Autodesk Inventor part; units mm, degrees
(part 2 of 2)
sketch "Sketch3" plane through (0.0295, 41.5, 0) normal (0, 1, 0) x (1, 0, 0)
  line L0 (1770.5478, -680) -> (1790.5478, -680)
  line L1 (1790.5478, -640) -> (1770.5478, -640)
  line L2 (1790.5478, -620) -> (1790.5478, -640)
  line L3 (1770.5478, -640) -> (1770.5478, -620)
  line L4 (1770.5478, -620) -> (1790.5478, -620)
  line L5 (1790.5478, -680) -> (1790.5478, -700)
  line L6 (1770.5478, -700) -> (1770.5478, -680)
  line L7 (1790.5478, -700) -> (1770.5478, -700)
  line L8 (1770.5478, -740) -> (1790.5478, -740)
  line L9 (1790.5478, -740) -> (1790.5478, -760)
  line L10 (1790.5478, -760) -> (1770.5478, -760)
  line L11 (1770.5478, -760) -> (1770.5478, -740)
  line L12 (1790.5478, -580) -> (1770.5478, -580)
  line L13 (1770.5478, -580) -> (1770.5478, -560)
  line L14 (1770.5478, -560) -> (1790.5478, -560)
  line L15 (1790.5478, -340) -> (1770.5478, -340)
  line L16 (1790.5478, -320) -> (1790.5478, -340)
  line L17 (1770.5478, -340) -> (1770.5478, -320)
  line L18 (1770.5478, -320) -> (1790.5478, -320)
  line L19 (1790.5478, -280) -> (1770.5478, -280)
  line L20 (1770.5478, -280) -> (1770.5478, -260)
  line L21 (1770.5478, -260) -> (1790.5478, -260)
  line L22 (1790.5478, -260) -> (1790.5478, -280)
  line L23 (1790.5478, -560) -> (1790.5478, -580)
  line L24 (1770.5478, -520) -> (1770.5478, -500)
  line L25 (1770.5478, -500) -> (1790.5478, -500)
  line L26 (1790.5478, -500) -> (1790.5478, -520)
  line L27 (1790.5478, -520) -> (1770.5478, -520)
  line L28 (1770.5478, -460) -> (1770.5478, -440)
  line L29 (1790.5478, -460) -> (1770.5478, -460)
  line L30 (1770.5478, -440) -> (1790.5478, -440)
  line L31 (1790.5478, -400) -> (1770.5478, -400)
  line L32 (1770.5478, -400) -> (1770.5478, -380)
  line L33 (1790.5478, -380) -> (1790.5478, -400)
  line L34 (1790.5478, -440) -> (1790.5478, -460)
  line L35 (1790.5478, -220) -> (1770.5478, -220)
  line L36 (1770.5478, -220) -> (1770.5478, -200)
  line L37 (1770.5478, -200) -> (1790.5478, -200)
  line L38 (1790.5478, -200) -> (1790.5478, -220)
  line L39 (1770.5478, -380) -> (1790.5478, -380)
  line L40 (1790.5478, -100) -> (1770.5478, -100)
  line L41 (1790.5478, -80) -> (1790.5478, -100)
  line L42 (1770.5478, -100) -> (1770.5478, -80)
  line L43 (1770.5478, -80) -> (1790.5478, -80)
  line L44 (1790.5478, -40) -> (1770.5478, -40)
  line L45 (1770.5478, -20) -> (1790.5478, -20)
  line L46 (1790.5478, -20) -> (1790.5478, -40)
  line L47 (1770.5478, -40) -> (1770.5478, -20)
  line L48 (1790.5478, -160) -> (1770.5478, -160)
  line L49 (1790.5478, -140) -> (1790.5478, -160)
  line L50 (1770.5478, -160) -> (1770.5478, -140)
  line L51 (1770.5478, -140) -> (1790.5478, -140)
  line L52 (1938.8211, -400) -> (1938.8211, -380)
  line L53 (1958.8211, -400) -> (1938.8211, -400)
  line L54 (1958.8211, -380) -> (1958.8211, -400)
  line L55 (1938.8211, -380) -> (1958.8211, -380)
  line L56 (1938.8211, -340) -> (1938.8211, -320)
  line L57 (1958.8211, -340) -> (1938.8211, -340)
  line L58 (1958.8211, -320) -> (1958.8211, -340)
  line L59 (1938.8211, -320) -> (1958.8211, -320)
  line L60 (1958.8211, -280) -> (1938.8211, -280)
  line L61 (1958.8211, -260) -> (1958.8211, -280)
  line L62 (1938.8211, -280) -> (1938.8211, -260)
  line L63 (1938.8211, -260) -> (1958.8211, -260)
  line L64 (1958.8211, -220) -> (1938.8211, -220)
  line L65 (1958.8211, -200) -> (1958.8211, -220)
  line L66 (1938.8211, -200) -> (1958.8211, -200)
  line L67 (1938.8211, -220) -> (1938.8211, -200)
  line L68 (1938.8211, -100) -> (1938.8211, -80)
  line L69 (1958.8211, -80) -> (1958.8211, -100)
  line L70 (1958.8211, -100) -> (1938.8211, -100)
  line L71 (1938.8211, -160) -> (1938.8211, -140)
  line L72 (1938.8211, -140) -> (1958.8211, -140)
  line L73 (1958.8211, -160) -> (1938.8211, -160)
  line L74 (1958.8211, -140) -> (1958.8211, -160)
  line L75 (1938.8211, -80) -> (1958.8211, -80)
  line L76 (1958.8211, -40) -> (1938.8211, -40)
  line L77 (1958.8211, -20) -> (1958.8211, -40)
  line L78 (1938.8211, -20) -> (1958.8211, -20)
  line L79 (1938.8211, -40) -> (1938.8211, -20)
  line L80 (1958.8211, -520) -> (1938.8211, -520)
  line L81 (1938.8211, -520) -> (1938.8211, -500)
  line L82 (1958.8211, -500) -> (1958.8211, -520)
  line L83 (1938.8211, -500) -> (1958.8211, -500)
  line L84 (1958.8211, -460) -> (1938.8211, -460)
  line L85 (1958.8211, -440) -> (1958.8211, -460)
  line L86 (1938.8211, -440) -> (1958.8211, -440)
  line L87 (1938.8211, -460) -> (1938.8211, -440)
  line L88 (1958.8211, -640) -> (1938.8211, -640)
  line L89 (1938.8211, -560) -> (1958.8211, -560)
  line L90 (1938.8211, -580) -> (1938.8211, -560)
  line L91 (1958.8211, -560) -> (1958.8211, -580)
  line L92 (1958.8211, -580) -> (1938.8211, -580)
  line L93 (1938.8211, -620) -> (1958.8211, -620)
  line L94 (1938.8211, -640) -> (1938.8211, -620)
  line L95 (1958.8211, -620) -> (1958.8211, -640)
  line L96 (1938.8211, -760) -> (1938.8211, -740)
  line L97 (1938.8211, -700) -> (1938.8211, -680)
  line L98 (1938.8211, -680) -> (1958.8211, -680)
  line L99 (1958.8211, -680) -> (1958.8211, -700)
  line L100 (1958.8211, -700) -> (1938.8211, -700)
  line L101 (1938.8211, -740) -> (1958.8211, -740)
  line L102 (1958.8211, -740) -> (1958.8211, -760)
  line L103 (1958.8211, -760) -> (1938.8211, -760)
  point P0 (-0.0295, 0)
  point P1 (1780.5478, -640)
  point P2 (1780.5478, -700)
  point P3 (1780.5478, -760)
  point P4 (1780.5478, -740)
  point P5 (1780.5478, -580)
  point P6 (1780.5478, -340)
  point P7 (1780.5478, -280)
  point P8 (1780.5478, -520)
  point P9 (1780.5478, -500)
  point P10 (1780.5478, -460)
  point P11 (1780.5478, -400)
  point P12 (1780.5478, -220)
  point P13 (1780.5478, -40)
  point P14 (1780.5478, -160)
  point P15 (1780.5478, -100)
  point P16 (1948.8211, -400)
  point P17 (1948.8211, -340)
  point P18 (1948.8211, -280)
  point P19 (1948.8211, -220)
  point P20 (1948.8211, -100)
  point P21 (1948.8211, -160)
  point P22 (1948.8211, -40)
  point P23 (1948.8211, -520)
  point P24 (1948.8211, -500)
  point P25 (1948.8211, -460)
  point P26 (1948.8211, -640)
  point P27 (1948.8211, -580)
  point P28 (1948.8211, -700)
  point P29 (1948.8211, -760)
  point P30 (1948.8211, -740)
  dimension "d459" = 20
  dimension "d460" = 20
  dimension "d461" = 20
  dimension "d462" = 20
  dimension "d463" = 20
  dimension "d464" = 20
  dimension "d465" = 20
  dimension "d466" = 20
  dimension "d467" = 20
  dimension "d468" = 20
  dimension "d469" = 20
  dimension "d470" = 20
  dimension "d471" = 20
  dimension "d472" = 20
  dimension "d473" = 20
  dimension "d474" = 20
  dimension "d475" = 20
  dimension "d476" = 20
  dimension "d477" = 20
  dimension "d478" = 20
  dimension "d479" = 20
  dimension "d480" = 20
  dimension "d481" = 40
  dimension "d482" = 40
  dimension "d483" = 40
  dimension "d484" = 40
  dimension "d485" = 40
  dimension "d486" = 40
  dimension "d487" = 40
  dimension "d488" = 40
  dimension "d489" = 40
  dimension "d490" = 20
  dimension "d491" = 20
  dimension "d492" = 40
  dimension "d493" = 20
  dimension "d494" = 20
  dimension "d495" = 40
  dimension "d496" = 20
  dimension "d497" = 20
  dimension "d498" = 20
  dimension "d499" = 20
  dimension "d500" = 20
  dimension "d501" = 20
  dimension "d502" = 20
  dimension "d503" = 20
  dimension "d504" = 20
  dimension "d505" = 20
  dimension "d506" = 20
  dimension "d507" = 20
  dimension "d508" = 20
  dimension "d509" = 20
  dimension "d510" = 20
  dimension "d511" = 20
  dimension "d512" = 20
  dimension "d513" = 20
  dimension "d514" = 20
  dimension "d515" = 20
  dimension "d516" = 20
  dimension "d517" = 20
  dimension "d518" = 40
  dimension "d519" = 40
  dimension "d520" = 40
  dimension "d521" = 40
  dimension "d522" = 40
  constraints: 208 end point, 52 parallel, 30 midpoint, 26 horizontal, 26 perpendicular
  measures "d459" distance from line of point (1780.548, -40) L45
  measures "d460" distance between parallel lines of L46 L47
  measures "d461" distance from line of point (1780.548, -100) L43
  measures "d462" distance between parallel lines of L41 L42
  measures "d463" distance from line of point (1780.548, -160) L51
  measures "d464" distance between parallel lines of L49 L50
  measures "d465" distance from line of point (1780.548, -220) L37
  measures "d466" distance between parallel lines of L38 L36
  measures "d467" distance from line of point (1780.548, -400) L39
  measures "d468" distance between parallel lines of L33 L32
  measures "d469" distance from line of point (1780.548, -460) L30
  measures "d470" distance between parallel lines of L34 L28
  measures "d471" distance from line of point (1780.548, -520) L25
  measures "d472" distance between parallel lines of L26 L24
  measures "d473" distance from line of point (1780.548, -580) L14
  measures "d474" distance between parallel lines of L23 L13
  measures "d475" distance from line of point (1780.548, -640) L4
  measures "d476" distance between parallel lines of L2 L3
  measures "d477" distance from line of point (1780.548, -700) L0
  measures "d478" distance between parallel lines of L5 L6
  measures "d479" distance from line of point (1780.548, -760) L8
  measures "d480" distance between parallel lines of L9 L11
  measures "d481" distance between parallel lines of L43 L44
  measures "d482" distance between parallel lines of L51 L40
  measures "d483" distance between parallel lines of L37 L48
  measures "d484" distance from line of point (1780.548, -740) L7
  measures "d485" distance between parallel lines of L0 L1
  measures "d486" distance between parallel lines of L4 L12
  measures "d487" distance between parallel lines of L14 L27
  measures "d488" distance from line of point (1780.548, -500) L29
  measures "d489" distance between parallel lines of L31 L30
  measures "d490" distance from line of point (1780.548, -280) L21
  measures "d491" distance between parallel lines of L22 L20
  measures "d492" distance between parallel lines of L21 L35
  measures "d493" distance from line of point (1780.548, -340) L18
  measures "d494" distance between parallel lines of L16 L17
  measures "d495" distance between parallel lines of L18 L19
  measures "d496" distance from line of point (1948.821, -40) L78
  measures "d497" distance between parallel lines of L77 L79
  measures "d498" distance from line of point (1948.821, -100) L75
  measures "d499" distance between parallel lines of L69 L68
  measures "d500" distance from line of point (1948.821, -160) L72
  measures "d501" distance between parallel lines of L74 L71
  measures "d502" distance from line of point (1948.821, -220) L66
  measures "d503" distance between parallel lines of L65 L67
  measures "d504" distance from line of point (1948.821, -400) L55
  measures "d505" distance between parallel lines of L54 L52
  measures "d506" distance from line of point (1948.821, -460) L86
  measures "d507" distance between parallel lines of L85 L87
  measures "d508" distance from line of point (1948.821, -520) L83
  measures "d509" distance between parallel lines of L82 L81
  measures "d510" distance from line of point (1948.821, -580) L89
  measures "d511" distance between parallel lines of L91 L90
  measures "d512" distance from line of point (1948.821, -640) L93
  measures "d513" distance between parallel lines of L95 L94
  measures "d514" distance from line of point (1948.821, -700) L98
  measures "d515" distance between parallel lines of L99 L97
  measures "d516" distance from line of point (1948.821, -760) L101
  measures "d517" distance between parallel lines of L102 L96
  measures "d518" distance between parallel lines of L75 L76
  measures "d519" distance between parallel lines of L72 L70
  measures "d520" distance between parallel lines of L66 L73
  measures "d521" distance from line of point (1948.821, -740) L100
  measures "d522" distance between parallel lines of L98 L88
extrude "Extrusion3" cut sketch "Sketch3" against normal through all
body "Solid1"
